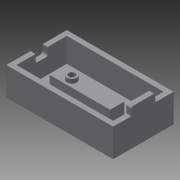
# Autodesk Inventor part: V2_unterteil
Saved by Autodesk Inventor 2015 (Build 190159000, 159)
## iProperties
Created: 2015-05-04
Part Number: V2_unterteil
Material: Generisch
Document SubType Name: Modeling
Designer: krumms
Density: 1 g/cm^3
Appearance: Vorgabe
Author: krumms
Autodesk Inventor part; units mm, degrees
ref_plane "YZ Plane" through (0, 0, 0) normal (1, 0, 0) x (0, 1, 0)
ref_plane "XZ Plane" through (0, 0, 0) normal (0, 1, 0) x (-1, 0, 0)
ref_plane "XY Plane" through (0, 0, 0) normal (0, 0, 1) x (1, 0, 0)
sketch "Skizze1" plane through (0, 0, 0) normal (0, 0, 1) x (1, 0, 0)
  line L0 (0, 0) -> (53, 0)
  line L1 (53, 0) -> (53, 30)
  line L2 (53, 30) -> (0, 30)
  line L3 (0, 30) -> (0, 0)
  dimension "d0" = 30
  dimension "d1" = 53
  constraints: 8 end point, 2 parallel, 1 horizontal, 1 perpendicular
  measures "d0" distance of L2.end L0.start
  measures "d1" distance of L0.start L0.end
extrude "Extrusion1" add sketch "Skizze1" along normal blind 2
sketch "Skizze2" plane through (0, 0, 2) normal (0, 0, 1) x (1, 0, 0)
  line L0 (0, 0) -> (53, 0)
  line L1 (53, 0) -> (53, 30)
  line L2 (53, 30) -> (0, 30)
  line L3 (0, 30) -> (0, 0)
  line L4 (2.5, 2.5) -> (50.5, 2.5)
  line L5 (50.5, 2.5) -> (50.5, 27.5)
  line L6 (50.5, 27.5) -> (2.5, 27.5)
  line L7 (2.5, 27.5) -> (2.5, 2.5)
  dimension "d4" = 25
  dimension "d5" = 48
  dimension "d6" = 2.5
  dimension "d7" = 2.5
  dimension "d8" = 2.5
  dimension "d9" = 2.5
  constraints: 16 end point, 4 parallel, 2 horizontal, 2 perpendicular
  measures "d4" distance of L6.end L4.start
  measures "d5" distance of L4.start L4.end
  measures "d6" distance between parallel lines of L3 L7
  measures "d7" distance between parallel lines of L1 L5
  measures "d8" distance between parallel lines of L0 L4
  measures "d9" distance between parallel lines of L2 L6
extrude "Extrusion2" add sketch "Skizze2" along normal blind 12
sketch "Skizze3" plane through (0, 0, 2) normal (0, 0, 1) x (1, 0, 0)
  line L0 (10, 18.5) -> (40, 18.5)
  line L1 (40, 18.5) -> (40, 11.5)
  line L2 (40, 11.5) -> (10, 11.5)
  line L3 (10, 11.5) -> (10, 18.5)
  line L4 (0, 30) -> (0, 0) projected
  line L5 (50.5, 27.5) -> (2.5, 27.5) projected
  line L6 (2.5, 2.5) -> (50.5, 2.5) projected
  dimension "d12" = 10
  dimension "d13" = 30
  dimension "d14" = 7
  dimension "d15" = 9
  dimension "d16" = 9
  constraints: 8 end point, 2 parallel, 1 horizontal, 1 perpendicular
  measures "d12" distance between parallel lines of L4 L3
  measures "d13" distance between parallel lines of L3 L1
  measures "d14" distance between parallel lines of L2 L0
  measures "d15" distance between parallel lines of L5 L0
  measures "d16" distance between parallel lines of L6 L2
extrude "Extrusion3" add sketch "Skizze3" along normal blind 7
hole "Bohrung1" at (17.5, 15, 9) direction (0, 0, -1) diameter 3.2 end through all
sketch "Skizze4" plane through (0, 0, 0) normal (0, 0, -1) x (-1, 0, 0)
  line L0 (-19.3149, 18.0854) -> (-15.7355, 18.1144)
  line L1 (-15.7355, 18.1144) -> (-13.9205, 15.0291)
  line L2 (-13.9205, 15.0291) -> (-15.6851, 11.9146)
  line L3 (-15.6851, 11.9146) -> (-19.2645, 11.8856)
  line L4 (-19.2645, 11.8856) -> (-21.0795, 14.9709)
  line L5 (-21.0795, 14.9709) -> (-19.3149, 18.0854)
  line L6 (-2.5, 2.5) -> (-50.5, 2.5) projected
  line L7 (-2.5, 27.5) -> (-2.5, 2.5) projected
  point P0 (0, 0)
  point P1 (-17.5, 15)
  dimension "d28" = 6.2
  dimension "d29" = 12.5
  dimension "d30" = 15
  constraints: 12 end point, 13 other
  measures "d28" distance between parallel lines of L3 L0
  measures "d29" distance from line of L6 point (-17.5, 15)
  measures "d30" distance from line of point (-17.5, 15) L7
extrude "Extrusion4" cut sketch "Skizze4" against normal blind 5
sketch "Skizze5" plane through (0, 0, 9) normal (0, 0, 1) x (1, 0, 0)
  circle A0 centre (17.5, 15) radius 2.5
  line L0 (2.5, 2.5) -> (2.5, 27.5) projected
  line L1 (40, 18.5) -> (10, 18.5) projected
  circle A1 centre (17.5, 15) radius 1.6
  point P0 (0, 0)
  dimension "d33" = 5
  dimension "d34" = 15
  dimension "d35" = 3.5
  constraints: 2 centre point, 1 coincident
  measures "d33" diameter of A0
  measures "d34" distance from line of A0.centre L0
  measures "d35" distance from line of L1 A0.centre
extrude "Extrusion5" add sketch "Skizze5" along normal blind 2
sketch "Skizze6" plane through (0, 0, 14) normal (0, 0, 1) x (1, 0, 0)
  line L0 (50.5, 27.5) -> (50.5, 2.5) projected
  line L1 (53, 0) -> (53, 30) projected
  line L2 (50.5, 9) -> (53, 9)
  line L3 (53, 9) -> (53, 21)
  line L4 (53, 21) -> (50.5, 21)
  line L5 (50.5, 21) -> (50.5, 9)
  line L6 (0, 0) -> (53, 0) projected
  line L7 (53, 30) -> (0, 30) projected
  dimension "d38" = 12
  dimension "d39" = 9
  dimension "d40" = 9
  constraints: 8 end point, 2 parallel, 2 point on line, 1 horizontal, 1 perpendicular
  measures "d38" distance between parallel lines of L4 L2
  measures "d39" distance between parallel lines of L6 L2
  measures "d40" distance between parallel lines of L7 L4
extrude "Extrusion6" add sketch "Skizze6" along normal blind 4
sketch "Skizze7" plane through (0, 0, 14) normal (0, 0, 1) x (1, 0, 0)
  line L0 (0, 30) -> (0, 0) projected
  line L1 (2.5, 2.5) -> (2.5, 27.5) projected
  line L2 (0, 12) -> (2.5, 12)
  line L3 (2.5, 12) -> (2.5, 18)
  line L4 (2.5, 18) -> (0, 18)
  line L5 (0, 18) -> (0, 12)
  line L6 (0, 0) -> (53, 0) projected
  line L7 (53, 30) -> (0, 30) projected
  dimension "d43" = 6
  dimension "d44" = 12
  dimension "d45" = 12
  constraints: 8 end point, 2 parallel, 2 point on line, 1 horizontal, 1 perpendicular
  measures "d43" distance between parallel lines of L4 L2
  measures "d44" distance between parallel lines of L6 L2
  measures "d45" distance between parallel lines of L7 L4
extrude "Extrusion7" cut sketch "Skizze7" against normal blind 4
fillet "Rundung1" radius 1 4 edges at (51.75, 21, 18) (51.75, 9, 18) (1.25, 18, 10) (1.25, 12, 10)
